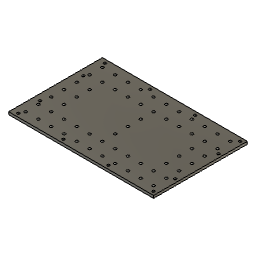
MFT Basic (Autodesk Fusion 360 design; units mm, degrees)
Autodesk Fusion 360 part; units mm, degrees
note: some values were not read from the file. Set by a fixed rule: which sketch regions a step uses.
sketch "Sketch1" plane through (0, 0, 0) normal (0, 0, 1) x (1, 0, 0)
  line L0 (544, -352) -> (-544, -352)
  line L1 (-544, -352) -> (-544, 352)
  line L2 (-544, 352) -> (544, 352)
  line L3 (544, 352) -> (544, -352)
  line L4 (544, -352) -> (-544, 352) construction
  line L5 (-544, -352) -> (544, 352) construction
  circle A0 centre (0, 0) radius 9.95
  circle A1 centre (-480, -288) radius 9.95
  circle A2 centre (-384, -288) radius 9.95
  circle A3 centre (-288, -288) radius 9.95
  circle A4 centre (-192, -288) radius 9.95
  circle A5 centre (-96, -288) radius 9.95
  circle A6 centre (0, -288) radius 9.95
  circle A7 centre (96, -288) radius 9.95
  circle A8 centre (192, -288) radius 9.95
  circle A9 centre (288, -288) radius 9.95
  circle A10 centre (384, -288) radius 9.95
  circle A11 centre (480, -288) radius 9.95
  circle A12 centre (-480, -192) radius 9.95
  circle A13 centre (-384, -192) radius 9.95
  circle A14 centre (-288, -192) radius 9.95
  circle A15 centre (-192, -192) radius 9.95
  circle A16 centre (-96, -192) radius 9.95
  circle A17 centre (0, -192) radius 9.95
  circle A18 centre (96, -192) radius 9.95
  circle A19 centre (192, -192) radius 9.95
  circle A20 centre (288, -192) radius 9.95
  circle A21 centre (384, -192) radius 9.95
  circle A22 centre (480, -192) radius 9.95
  circle A23 centre (-480, -96) radius 9.95
  circle A24 centre (-384, -96) radius 9.95
  circle A25 centre (0, -96) radius 9.95
  circle A26 centre (384, -96) radius 9.95
  circle A27 centre (480, -96) radius 9.95
  circle A28 centre (-480, 0) radius 9.95
  circle A29 centre (-384, 0) radius 9.95
  circle A30 centre (384, 0) radius 9.95
  circle A31 centre (480, 0) radius 9.95
  circle A32 centre (-480, 96) radius 9.95
  circle A33 centre (-384, 96) radius 9.95
  circle A34 centre (0, 96) radius 9.95
  circle A35 centre (384, 96) radius 9.95
  circle A36 centre (480, 96) radius 9.95
  circle A37 centre (-480, 192) radius 9.95
  circle A38 centre (-384, 192) radius 9.95
  circle A39 centre (-288, 192) radius 9.95
  circle A40 centre (-192, 192) radius 9.95
  circle A41 centre (-96, 192) radius 9.95
  circle A42 centre (0, 192) radius 9.95
  circle A43 centre (96, 192) radius 9.95
  circle A44 centre (192, 192) radius 9.95
  circle A45 centre (288, 192) radius 9.95
  circle A46 centre (384, 192) radius 9.95
  circle A47 centre (480, 192) radius 9.95
  circle A48 centre (-480, 288) radius 9.95
  circle A49 centre (-384, 288) radius 9.95
  circle A50 centre (-288, 288) radius 9.95
  circle A51 centre (-192, 288) radius 9.95
  circle A52 centre (-96, 288) radius 9.95
  circle A53 centre (0, 288) radius 9.95
  circle A54 centre (96, 288) radius 9.95
  circle A55 centre (192, 288) radius 9.95
  circle A56 centre (288, 288) radius 9.95
  circle A57 centre (384, 288) radius 9.95
  circle A58 centre (480, 288) radius 9.95
  dimension "d1" = 1088
  dimension "d2" = 704
  dimension "d3" = 19.9
  dimension "d6" = 96
  dimension "d7" = 96
  constraint horizontal L0
  constraint perpendicular L0 L1
  constraint parallel L0 L2
  constraint parallel L1 L3
  constraint coincident L4 A0.centre
  constraint coincident L5 A0.centre
  constraint coincident A0.centre origin
  measures "d1" distance of L1.end L2.end
  measures "d2" distance of L0.end L1.end
  measures "d3" diameter of A0
extrude "Extrude1" add sketch "Sketch1" along normal blind 19.05
sketch "Sketch2" plane through (0, 0, 19.05) normal (0, 0, 1) x (-1, 0, 0)
  circle A0 centre (192, -192) radius 9.95
  circle A1 centre (-480, 0) radius 9.95
  circle A2 centre (-384, -288) radius 9.95
  circle A3 centre (480, -192) radius 9.95
  circle A4 centre (480, -96) radius 9.95
  circle A5 centre (96, -192) radius 9.95
  circle A6 centre (384, -192) radius 9.95
  circle A7 centre (288, -192) radius 9.95
  circle A8 centre (96, 288) radius 9.95
  circle A9 centre (0, 0) radius 9.95
  circle A10 centre (-96, 288) radius 9.95
  circle A11 centre (384, 288) radius 9.95
  circle A12 centre (288, 288) radius 9.95
  circle A13 centre (0, 288) radius 9.95
  circle A14 centre (192, 288) radius 9.95
  circle A15 centre (480, 288) radius 9.95
  circle A16 centre (-192, 288) radius 9.95
  circle A17 centre (-384, 288) radius 9.95
  circle A18 centre (384, -288) radius 9.95
  circle A19 centre (-96, -288) radius 9.95
  circle A20 centre (480, -288) radius 9.95
  circle A21 centre (96, -288) radius 9.95
  circle A22 centre (192, -288) radius 9.95
  circle A23 centre (-480, -96) radius 9.95
  circle A24 centre (288, -288) radius 9.95
  circle A25 centre (-480, -192) radius 9.95
  circle A26 centre (0, -288) radius 9.95
  circle A27 centre (-384, -192) radius 9.95
  circle A28 centre (-192, -288) radius 9.95
  circle A29 centre (-480, 288) radius 9.95
  circle A30 centre (384, 192) radius 9.95
  circle A31 centre (480, 192) radius 9.95
  circle A32 centre (288, 192) radius 9.95
  circle A33 centre (96, 192) radius 9.95
  circle A34 centre (192, 192) radius 9.95
  circle A35 centre (0, 192) radius 9.95
  circle A36 centre (-192, 192) radius 9.95
  circle A37 centre (-96, 192) radius 9.95
  circle A38 centre (-288, 192) radius 9.95
  circle A39 centre (-480, 192) radius 9.95
  circle A40 centre (480, 96) radius 9.95
  circle A41 centre (0, 96) radius 9.95
  circle A42 centre (384, 96) radius 9.95
  circle A43 centre (-384, 0) radius 9.95
  circle A44 centre (-480, 96) radius 9.95
  circle A45 centre (384, 0) radius 9.95
  circle A46 centre (-384, 96) radius 9.95
  circle A47 centre (480, 0) radius 9.95
  circle A48 centre (384, -96) radius 9.95
  circle A49 centre (0, -96) radius 9.95
  circle A50 centre (-384, -96) radius 9.95
  circle A51 centre (-480, -288) radius 9.95
  circle A52 centre (-288, -192) radius 9.95
  circle A53 centre (-384, 192) radius 9.95
  circle A54 centre (-288, -288) radius 9.95
  circle A55 centre (-192, -192) radius 9.95
  circle A56 centre (-288, 288) radius 9.95
  circle A57 centre (-96, -192) radius 9.95
  circle A58 centre (0, -192) radius 9.95
  line L0 (-544, -352) -> (544, -352)
  line L1 (544, -352) -> (544, 352)
  line L2 (544, 352) -> (-544, 352)
  line L3 (-544, 352) -> (-544, -352)
  point P0 (497.95, -325)
  point P1 (159.6333, -325)
  point P2 (-178.6833, -325)
  point P3 (-517, -325)
  point P4 (497.95, -162.5)
  point P5 (-517, -162.5)
  point P6 (-517, 0)
  point P7 (497.95, 162.5)
  point P8 (-517, 162.5)
  point P9 (497.95, 325)
  point P10 (159.6333, 325)
  point P11 (-178.6833, 325)
  point P12 (-517, 325)
  dimension "d10" = 46.05
  dimension "d11" = 27
  dimension "d14" = -1014.95
  dimension "d15" = 650
  measures "d10" distance of L1 P0
  measures "d11" distance of L0 P0
hole "Hole1" at (-497.95, 325, 19.05) at (-497.95, 162.5, 19.05) at (-497.95, -162.5, 19.05) at (-497.95, -325, 19.05) at (-159.6333, -325, 19.05) at (178.6833, -325, 19.05) at (517, -325, 19.05) at (517, -162.5, 19.05) at (517, 162.5, 19.05) at (517, 325, 19.05) at (178.6833, 325, 19.05) at (-159.6333, 325, 19.05) direction (0, 0, -1) diameter 6.35 depth 254 tip angle 180 counterbore diameter 19.05 counterbore depth 9.8425
